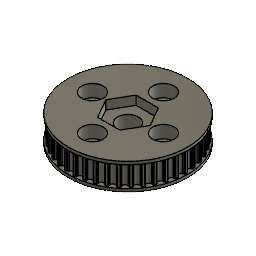
grt_cardan_joint_pulley_42T_20190328 (Autodesk Fusion 360 design; units mm, degrees)
Autodesk Fusion 360 part; units mm, degrees
(part 1 of 2)
sketch "Skizze1" plane through (0, 0, 0) normal (0, 1, 0) x (1, 0, 0)
  line L0 (0, 20.9325) -> (0, 0) construction
  arc A0 (-0.7739, 19.0309) -> (0, 18.5325) centre (0, 19.3825) ccw
  arc A1 (-0.8921, 19.4273) -> (-0.7739, 19.0309) centre (0.61, 19.6597) ccw
  arc A2 (-0.8921, 19.4273) -> (-1.1539, 19.6387) centre (-1.1392, 19.3891) ccw
  arc A3 (0, 20.5515) -> (-1.5358, 20.4941) centre (0, 0) ccw construction
  arc A4 (-1.1539, 19.6387) -> (-1.4701, 19.6175) centre (0, 0) ccw
  arc A5 (0, 20.9325) -> (-1.5643, 20.874) centre (0, 0) ccw construction
  line L1 (0, 0) -> (-1.5643, 20.874) construction
  line L2 (-1.4701, 19.6175) -> (0, 0)
  line L3 (0, 18.5325) -> (0, 0)
  dimension "d2" = 1.14
  dimension "d4" = 0.85
  dimension "d5" = 1.52
  dimension "d6" = 0.25
  dimension "d7" = 0.61
  dimension "d8" = 0.381
  dimension "d12" = 1.26
  dimension "d19" = 4.286
  dimension "d23" = 19.6725
  dimension "d24" = 2.4
  measures "d4" radius of A0
  measures "d5" radius of A1
  measures "d6" radius of A2
  measures "d19" angle of L0 L1
  measures "d23" distance of L0.end
  measures "d24" distance of L0.end
extrude "Extrusion1" add sketch "Skizze1" along normal blind 7 makes body 1
mirror "Spiegeln1" about plane through (0, 0, -18.5325) normal (1, 0, 0) of bodies 1 makes body 2
combine "Kombinieren1" operation add target body 1 tool bodies 2
pattern_circular "C-Anordnung1" count 42 over 360 about axis through (0, 1.75, 0) along (0, 1, 0) of bodies 1 makes body 3 at (-0.9801, 2.3333, -13.0783) makes body 4 at (-4.4504, 0, -12.0378) makes body 5 at (-6.1948, 0, -11.2401) makes body 6 at (-6.6368, 0, -10.9849) makes body 7 at (-8.1999, 0, -9.873) makes body 8 at (-9.5798, 7, -8.5406) makes body 9 at (-10.7457, 0, -7.0175) makes body 10 at (-11.6716, 0, -5.3375) makes body 11 at (-12.6502, 0, -2.1648) makes body 12 at (-12.7263, 0, -1.6601) makes body 13 at (-12.8316, 0, 0.2552) makes body 14 at (-12.6502, 0, 2.1648) makes body 15 at (-11.6716, 0, 5.3375) makes body 16 at (-10.7457, 0, 7.0175) makes body 17 at (-9.5798, 0, 8.5406) makes body 18 at (-9.2327, 7, 8.9148) makes body 19 at (-7.8009, 0, 10.1912) makes body 20 at (-4.9254, 0, 11.8514) makes body 21 at (-4.4504, 0, 12.0378) makes body 22 at (-1.2134, 0, 12.7766) makes body 23 at (-0.7044, 0, 12.8148) makes body 24 at (1.2134, 0, 12.7766) makes body 25 at (4.4504, 0, 12.0378) makes body 26 at (4.9254, 0, 11.8514) makes body 27 at (6.6368, 0, 10.9849) makes body 28 at (9.2327, 0, 8.9148) makes body 29 at (10.4582, 0, 7.4391) makes body 30 at (10.7457, 0, 7.0175) makes body 31 at (11.6716, 7, 5.3375) makes body 32 at (12.3367, 0, 3.5383) makes body 33 at (12.7263, 0, 1.6601) makes body 34 at (12.8316, 0, -0.2552) makes body 35 at (12.6502, 0, -2.1648) makes body 36 at (11.6716, 0, -5.3375) makes body 37 at (11.4502, 0, -5.7973) makes body 38 at (10.4582, 0, -7.4391) makes body 39 at (9.2327, 0, -8.9148) makes body 40 at (7.8009, 0, -10.1912) makes body 41 at (6.1948, 0, -11.2401) makes body 42 at (4.4504, 0, -12.0378) makes body 43 at (0.9801, 2.3333, -13.0783)
combine "Kombinieren2" operation add target body 1 tool bodies 21 20 19 3 18 17 8 15 7 12 9 11 10 16 6 5 14 4 13 41 31 39 27 22 23 29 25 24 26 42 28 43 30 38 34 33 37 32 36 35 40
sketch "Skizze2" plane through (0, 7, 0) normal (0, 1, 0) x (-1, 0, 0)
  arc A0 (-1.786, -19.5913) -> (-1.1539, -19.6387) centre (0, 0) ccw
  arc A1 (-1.1539, -19.6387) -> (-0.8921, -19.4273) centre (-1.1392, -19.3891) ccw
  arc A2 (-0.7739, -19.0309) -> (-0.8921, -19.4273) centre (0.61, -19.6597) ccw
  arc A3 (0.7739, -19.0309) -> (-0.7739, -19.0309) centre (0, -19.3825) ccw
  arc A4 (0.8921, -19.4273) -> (0.7739, -19.0309) centre (-0.61, -19.6597) ccw
  arc A5 (0.8921, -19.4273) -> (1.1539, -19.6387) centre (1.1392, -19.3891) ccw
  arc A6 (1.1539, -19.6387) -> (1.786, -19.5913) centre (0, 0) ccw
  arc A7 (1.786, -19.5913) -> (2.0133, -19.3433) centre (1.7633, -19.3423) ccw
  arc A8 (2.0712, -18.9337) -> (2.0133, -19.3433) centre (3.5333, -19.3492) ccw
  arc A9 (3.6017, -18.703) -> (2.0712, -18.9337) centre (2.8888, -19.166) ccw
  arc A10 (3.7777, -19.0773) -> (3.6017, -18.703) centre (2.3269, -19.531) ccw
  arc A11 (3.7777, -19.0773) -> (4.068, -19.2473) centre (4.0163, -19.0027) ccw
  arc A12 (4.068, -19.2473) -> (4.686, -19.1063) centre (0, 0) ccw
  arc A13 (4.686, -19.1063) -> (4.8738, -18.8272) centre (4.6264, -18.8635) ccw
  arc A14 (4.87, -18.4136) -> (4.8738, -18.8272) centre (6.3777, -18.6064) ccw
  arc A15 (6.349, -17.9573) -> (4.87, -18.4136) centre (5.7131, -18.5214) ccw
  arc A16 (6.5788, -18.3012) -> (6.349, -17.9573) centre (5.2119, -18.966) ccw
  arc A17 (6.5788, -18.3012) -> (6.8912, -18.4261) centre (6.8036, -18.1919) ccw
  arc A18 (6.8912, -18.4261) -> (7.4813, -18.1945) centre (0, 0) ccw
  arc A19 (7.4813, -18.1945) -> (7.6254, -17.8905) centre (7.3862, -17.9632) ccw
  arc A20 (7.56, -17.4821) -> (7.6254, -17.8905) centre (9.0796, -17.4481) ccw
  arc A21 (8.9545, -16.8105) -> (7.56, -17.4821) centre (8.4098, -17.463) ccw
  arc A22 (9.233, -17.1163) -> (8.9545, -16.8105) centre (7.9804, -17.9774) ccw
  arc A23 (9.233, -17.1163) -> (9.5605, -17.1932) centre (9.439, -16.9747) ccw
  arc A24 (9.5605, -17.1932) -> (10.1095, -16.8762) centre (0, 0) ccw
  arc A25 (10.1095, -16.8762) -> (10.2067, -16.5541) centre (9.981, -16.6617) ccw
  arc A26 (10.0811, -16.16) -> (10.2067, -16.5541) centre (11.5787, -15.8999) ccw
  arc A27 (11.3599, -15.2882) -> (10.0811, -16.16) centre (10.9186, -16.0146) ccw
  arc A28 (11.6809, -15.549) -> (11.3599, -15.2882) centre (10.5707, -16.5872) ccw
  arc A29 (11.6809, -15.549) -> (12.0162, -15.5762) centre (11.8635, -15.3783) ccw
  arc A30 (12.0162, -15.5762) -> (12.5118, -15.181) centre (0, 0) ccw
  arc A31 (12.5118, -15.181) -> (12.5599, -14.848) centre (12.3528, -14.9881) ccw
  arc A32 (12.377, -14.477) -> (12.5599, -14.848) centre (13.8191, -13.9966) ccw
  arc A33 (13.5116, -13.4243) -> (12.377, -14.477) centre (13.1835, -14.2084) ccw
  arc A34 (13.8679, -13.6344) -> (13.5116, -13.4243) centre (12.9248, -14.8264) ccw
  arc A35 (13.8679, -13.6344) -> (14.2035, -13.6113) centre (14.023, -13.4384) ccw
  arc A36 (14.2035, -13.6113) -> (14.6347, -13.1466) centre (0, 0) ccw
  arc A37 (14.6347, -13.1466) -> (14.6326, -12.8102) centre (14.4487, -12.9796) ccw
  arc A38 (14.3965, -12.4706) -> (14.6326, -12.8102) centre (15.7509, -11.7807) ccw
  arc A39 (15.3615, -11.2606) -> (14.3965, -12.4706) centre (15.1539, -12.0848) ccw
  arc A40 (15.7451, -11.4152) -> (15.3615, -11.2606) centre (14.9902, -12.7345) ccw
  arc A41 (15.7451, -11.4152) -> (16.0735, -11.3424) centre (15.8693, -11.1982) ccw
  arc A42 (16.0735, -11.3424) -> (16.4306, -10.8186) centre (0, 0) ccw
  arc A43 (16.4306, -10.8186) -> (16.3785, -10.4863) centre (16.2218, -10.6811) ccw
  arc A44 (16.0943, -10.1857) -> (16.3785, -10.4863) centre (17.3308, -9.3015) ccw
  arc A45 (16.8682, -8.8453) -> (16.0943, -10.1857) centre (16.7858, -9.6913) ccw
  arc A46 (17.2706, -8.941) -> (16.8682, -8.8453) centre (16.7208, -10.3581) ccw
  arc A47 (17.2706, -8.941) -> (17.5845, -8.8201) centre (17.361, -8.708) ccw
  arc A48 (17.5845, -8.8201) -> (17.8596, -8.2489) centre (0, 0) ccw
  arc A49 (17.8596, -8.2489) -> (17.7584, -7.9281) centre (17.6326, -8.1441) ccw
  arc A50 (17.4327, -7.6732) -> (17.7584, -7.9281) centre (18.5235, -6.6146) ccw
  arc A51 (17.9981, -6.2324) -> (17.4327, -7.6732) centre (18.0427, -7.0812) ccw
  arc A52 (18.4103, -6.2671) -> (17.9981, -6.2324) centre (18.0778, -7.7503) ccw
  arc A53 (18.4103, -6.2671) -> (18.7027, -6.1007) centre (18.465, -6.0232) ccw
  arc A54 (18.7027, -6.1007) -> (18.8895, -5.4949) centre (0, 0) ccw
  arc A55 (18.8895, -5.4949) -> (18.7417, -5.1927) centre (18.6495, -5.4251) ccw
  arc A56 (18.3816, -4.9893) -> (18.7417, -5.1927) centre (19.3025, -3.78) ccw
  arc A57 (18.726, -3.4803) -> (18.3816, -4.9893) centre (18.8966, -4.313) ccw
  arc A58 (19.1387, -3.4532) -> (18.726, -3.4803) centre (19.031, -4.9694) ccw
  arc A59 (19.1387, -3.4532) -> (19.403, -3.2451) centre (19.1565, -3.2038) ccw
  arc A60 (19.403, -3.2451) -> (19.4975, -2.6182) centre (0, 0) ccw
  arc A61 (19.4975, -2.6182) -> (19.3063, -2.3414) centre (19.2497, -2.585) ccw
  arc A62 (18.9199, -2.1939) -> (19.3063, -2.3414) centre (19.6503, -0.8609) ccw
  arc A63 (19.0356, -0.6505) -> (18.9199, -2.1939) centre (19.3283, -1.4485) ccw
  arc A64 (19.4396, -0.5622) -> (19.0356, -0.6505) centre (19.5591, -2.0775) ccw
  arc A65 (19.4396, -0.5622) -> (19.67, -0.317) centre (19.42, -0.3129) ccw
  arc A66 (19.67, -0.317) -> (19.67, 0.317) centre (0, 0) ccw
  arc A67 (19.67, 0.317) -> (19.4396, 0.5622) centre (19.42, 0.3129) ccw
  arc A68 (19.0356, 0.6505) -> (19.4396, 0.5622) centre (19.5591, 2.0775) ccw
  arc A69 (18.9199, 2.1939) -> (19.0356, 0.6505) centre (19.3283, 1.4485) ccw
  arc A70 (19.3063, 2.3414) -> (18.9199, 2.1939) centre (19.6503, 0.8609) ccw
  arc A71 (19.3063, 2.3414) -> (19.4975, 2.6182) centre (19.2497, 2.585) ccw
  arc A72 (19.4975, 2.6182) -> (19.403, 3.2451) centre (0, 0) ccw
  arc A73 (19.403, 3.2451) -> (19.1387, 3.4532) centre (19.1565, 3.2038) ccw
  arc A74 (18.726, 3.4803) -> (19.1387, 3.4532) centre (19.031, 4.9694) ccw
  arc A75 (18.3816, 4.9893) -> (18.726, 3.4803) centre (18.8966, 4.313) ccw
  arc A76 (18.7417, 5.1927) -> (18.3816, 4.9893) centre (19.3025, 3.78) ccw
  arc A77 (18.7417, 5.1927) -> (18.8895, 5.4949) centre (18.6495, 5.4251) ccw
  arc A78 (18.8895, 5.4949) -> (18.7027, 6.1007) centre (0, 0) ccw
  arc A79 (18.7027, 6.1007) -> (18.4103, 6.2671) centre (18.465, 6.0232) ccw
  arc A80 (17.9981, 6.2324) -> (18.4103, 6.2671) centre (18.0778, 7.7503) ccw
  arc A81 (17.4327, 7.6732) -> (17.9981, 6.2324) centre (18.0427, 7.0812) ccw
  arc A82 (17.7584, 7.9281) -> (17.4327, 7.6732) centre (18.5235, 6.6146) ccw
  arc A83 (17.7584, 7.9281) -> (17.8596, 8.2489) centre (17.6326, 8.1441) ccw
  arc A84 (17.8596, 8.2489) -> (17.5845, 8.8201) centre (0, 0) ccw
  arc A85 (17.5845, 8.8201) -> (17.2706, 8.941) centre (17.361, 8.708) ccw
  arc A86 (16.8682, 8.8453) -> (17.2706, 8.941) centre (16.7208, 10.3581) ccw
  arc A87 (16.0943, 10.1857) -> (16.8682, 8.8453) centre (16.7858, 9.6913) ccw
  arc A88 (16.3785, 10.4863) -> (16.0943, 10.1857) centre (17.3308, 9.3015) ccw
  arc A89 (16.3785, 10.4863) -> (16.4306, 10.8186) centre (16.2218, 10.6811) ccw
  arc A90 (16.4306, 10.8186) -> (16.0735, 11.3424) centre (0, 0) ccw
  arc A91 (16.0735, 11.3424) -> (15.7451, 11.4152) centre (15.8693, 11.1982) ccw
  arc A92 (15.3615, 11.2606) -> (15.7451, 11.4152) centre (14.9902, 12.7345) ccw
  arc A93 (14.3965, 12.4706) -> (15.3615, 11.2606) centre (15.1539, 12.0848) ccw
  arc A94 (14.6326, 12.8102) -> (14.3965, 12.4706) centre (15.7509, 11.7807) ccw
  arc A95 (14.6326, 12.8102) -> (14.6347, 13.1466) centre (14.4487, 12.9796) ccw
  arc A96 (14.6347, 13.1466) -> (14.2035, 13.6113) centre (0, 0) ccw
  arc A97 (14.2035, 13.6113) -> (13.8679, 13.6344) centre (14.023, 13.4384) ccw
  arc A98 (13.5116, 13.4243) -> (13.8679, 13.6344) centre (12.9248, 14.8264) ccw
  arc A99 (12.377, 14.477) -> (13.5116, 13.4243) centre (13.1835, 14.2084) ccw
  arc A100 (12.5599, 14.848) -> (12.377, 14.477) centre (13.8191, 13.9966) ccw
  arc A101 (12.5599, 14.848) -> (12.5118, 15.181) centre (12.3528, 14.9881) ccw
  arc A102 (12.5118, 15.181) -> (12.0162, 15.5762) centre (0, 0) ccw
  arc A103 (12.0162, 15.5762) -> (11.6809, 15.549) centre (11.8635, 15.3783) ccw
  arc A104 (11.3599, 15.2882) -> (11.6809, 15.549) centre (10.5707, 16.5872) ccw
  arc A105 (10.0811, 16.16) -> (11.3599, 15.2882) centre (10.9186, 16.0146) ccw
  arc A106 (10.2067, 16.5541) -> (10.0811, 16.16) centre (11.5787, 15.8999) ccw
  arc A107 (10.2067, 16.5541) -> (10.1095, 16.8762) centre (9.981, 16.6617) ccw
  arc A108 (10.1095, 16.8762) -> (9.5605, 17.1932) centre (0, 0) ccw
  arc A109 (9.5605, 17.1932) -> (9.233, 17.1163) centre (9.439, 16.9747) ccw
  arc A110 (8.9545, 16.8105) -> (9.233, 17.1163) centre (7.9804, 17.9774) ccw
  arc A111 (7.56, 17.4821) -> (8.9545, 16.8105) centre (8.4098, 17.463) ccw
  arc A112 (7.6254, 17.8905) -> (7.56, 17.4821) centre (9.0796, 17.4481) ccw
  arc A113 (7.6254, 17.8905) -> (7.4813, 18.1945) centre (7.3862, 17.9632) ccw
  arc A114 (7.4813, 18.1945) -> (6.8912, 18.4261) centre (0, 0) ccw
  arc A115 (6.8912, 18.4261) -> (6.5788, 18.3012) centre (6.8036, 18.1919) ccw
  arc A116 (6.349, 17.9573) -> (6.5788, 18.3012) centre (5.2119, 18.966) ccw
  arc A117 (4.87, 18.4136) -> (6.349, 17.9573) centre (5.7131, 18.5214) ccw
  arc A118 (4.8738, 18.8272) -> (4.87, 18.4136) centre (6.3777, 18.6064) ccw
  arc A119 (4.8738, 18.8272) -> (4.686, 19.1063) centre (4.6264, 18.8635) ccw
  arc A120 (4.686, 19.1063) -> (4.068, 19.2473) centre (0, 0) ccw
  arc A121 (4.068, 19.2473) -> (3.7777, 19.0773) centre (4.0163, 19.0027) ccw
  arc A122 (3.6017, 18.703) -> (3.7777, 19.0773) centre (2.3269, 19.531) ccw
  arc A123 (2.0712, 18.9337) -> (3.6017, 18.703) centre (2.8888, 19.166) ccw
  arc A124 (2.0133, 19.3433) -> (2.0712, 18.9337) centre (3.5333, 19.3492) ccw
  arc A125 (2.0133, 19.3433) -> (1.786, 19.5913) centre (1.7633, 19.3423) ccw
  arc A126 (1.786, 19.5913) -> (1.1539, 19.6387) centre (0, 0) ccw
  arc A127 (1.1539, 19.6387) -> (0.8921, 19.4273) centre (1.1392, 19.3891) ccw
  arc A128 (0.7739, 19.0309) -> (0.8921, 19.4273) centre (-0.61, 19.6597) ccw
  arc A129 (-0.7739, 19.0309) -> (0.7739, 19.0309) centre (0, 19.3825) ccw
  arc A130 (-0.8921, 19.4273) -> (-0.7739, 19.0309) centre (0.61, 19.6597) ccw
  arc A131 (-0.8921, 19.4273) -> (-1.1539, 19.6387) centre (-1.1392, 19.3891) ccw
  arc A132 (-1.1539, 19.6387) -> (-1.786, 19.5913) centre (0, 0) ccw
  arc A133 (-1.786, 19.5913) -> (-2.0133, 19.3433) centre (-1.7633, 19.3423) ccw
  arc A134 (-2.0712, 18.9337) -> (-2.0133, 19.3433) centre (-3.5333, 19.3492) ccw
  arc A135 (-3.6017, 18.703) -> (-2.0712, 18.9337) centre (-2.8888, 19.166) ccw
  arc A136 (-3.7777, 19.0773) -> (-3.6017, 18.703) centre (-2.3269, 19.531) ccw
  arc A137 (-3.7777, 19.0773) -> (-4.068, 19.2473) centre (-4.0163, 19.0027) ccw
  arc A138 (-4.068, 19.2473) -> (-4.686, 19.1063) centre (0, 0) ccw
  arc A139 (-4.686, 19.1063) -> (-4.8738, 18.8272) centre (-4.6264, 18.8635) ccw
  arc A140 (-4.87, 18.4136) -> (-4.8738, 18.8272) centre (-6.3777, 18.6064) ccw
  arc A141 (-6.349, 17.9573) -> (-4.87, 18.4136) centre (-5.7131, 18.5214) ccw
  arc A142 (-6.5788, 18.3012) -> (-6.349, 17.9573) centre (-5.2119, 18.966) ccw
  arc A143 (-6.5788, 18.3012) -> (-6.8912, 18.4261) centre (-6.8036, 18.1919) ccw
  arc A144 (-6.8912, 18.4261) -> (-7.4813, 18.1945) centre (0, 0) ccw
  arc A145 (-7.4813, 18.1945) -> (-7.6254, 17.8905) centre (-7.3862, 17.9632) ccw
  arc A146 (-7.56, 17.4821) -> (-7.6254, 17.8905) centre (-9.0796, 17.4481) ccw
  arc A147 (-8.9545, 16.8105) -> (-7.56, 17.4821) centre (-8.4098, 17.463) ccw
  arc A148 (-9.233, 17.1163) -> (-8.9545, 16.8105) centre (-7.9804, 17.9774) ccw
  arc A149 (-9.233, 17.1163) -> (-9.5605, 17.1932) centre (-9.439, 16.9747) ccw
  arc A150 (-9.5605, 17.1932) -> (-10.1095, 16.8762) centre (0, 0) ccw
  arc A151 (-10.1095, 16.8762) -> (-10.2067, 16.5541) centre (-9.981, 16.6617) ccw
  arc A152 (-10.0811, 16.16) -> (-10.2067, 16.5541) centre (-11.5787, 15.8999) ccw
  arc A153 (-11.3599, 15.2882) -> (-10.0811, 16.16) centre (-10.9186, 16.0146) ccw
  arc A154 (-11.6809, 15.549) -> (-11.3599, 15.2882) centre (-10.5707, 16.5872) ccw
  arc A155 (-11.6809, 15.549) -> (-12.0162, 15.5762) centre (-11.8635, 15.3783) ccw
  arc A156 (-12.0162, 15.5762) -> (-12.5118, 15.181) centre (0, 0) ccw
  arc A157 (-12.5118, 15.181) -> (-12.5599, 14.848) centre (-12.3528, 14.9881) ccw
  arc A158 (-12.377, 14.477) -> (-12.5599, 14.848) centre (-13.8191, 13.9966) ccw
  arc A159 (-13.5116, 13.4243) -> (-12.377, 14.477) centre (-13.1835, 14.2084) ccw
  arc A160 (-13.8679, 13.6344) -> (-13.5116, 13.4243) centre (-12.9248, 14.8264) ccw
  arc A161 (-13.8679, 13.6344) -> (-14.2035, 13.6113) centre (-14.023, 13.4384) ccw
  arc A162 (-14.2035, 13.6113) -> (-14.6347, 13.1466) centre (0, 0) ccw
  arc A163 (-14.6347, 13.1466) -> (-14.6326, 12.8102) centre (-14.4487, 12.9796) ccw
  arc A164 (-14.3965, 12.4706) -> (-14.6326, 12.8102) centre (-15.7509, 11.7807) ccw
  arc A165 (-15.3615, 11.2606) -> (-14.3965, 12.4706) centre (-15.1539, 12.0848) ccw
  arc A166 (-15.7451, 11.4152) -> (-15.3615, 11.2606) centre (-14.9902, 12.7345) ccw
  arc A167 (-15.7451, 11.4152) -> (-16.0735, 11.3424) centre (-15.8693, 11.1982) ccw
  arc A168 (-16.0735, 11.3424) -> (-16.4306, 10.8186) centre (0, 0) ccw
  arc A169 (-16.4306, 10.8186) -> (-16.3785, 10.4863) centre (-16.2218, 10.6811) ccw
  arc A170 (-16.0943, 10.1857) -> (-16.3785, 10.4863) centre (-17.3308, 9.3015) ccw
  arc A171 (-16.8682, 8.8453) -> (-16.0943, 10.1857) centre (-16.7858, 9.6913) ccw
  arc A172 (-17.2706, 8.941) -> (-16.8682, 8.8453) centre (-16.7208, 10.3581) ccw
  arc A173 (-17.2706, 8.941) -> (-17.5845, 8.8201) centre (-17.361, 8.708) ccw
  arc A174 (-17.5845, 8.8201) -> (-17.8596, 8.2489) centre (0, 0) ccw
  arc A175 (-17.8596, 8.2489) -> (-17.7584, 7.9281) centre (-17.6326, 8.1441) ccw
  arc A176 (-17.4327, 7.6732) -> (-17.7584, 7.9281) centre (-18.5235, 6.6146) ccw
  arc A177 (-17.9981, 6.2324) -> (-17.4327, 7.6732) centre (-18.0427, 7.0812) ccw
  arc A178 (-18.4103, 6.2671) -> (-17.9981, 6.2324) centre (-18.0778, 7.7503) ccw
  arc A179 (-18.4103, 6.2671) -> (-18.7027, 6.1007) centre (-18.465, 6.0232) ccw
  arc A180 (-18.7027, 6.1007) -> (-18.8895, 5.4949) centre (0, 0) ccw
  arc A181 (-18.8895, 5.4949) -> (-18.7417, 5.1927) centre (-18.6495, 5.4251) ccw
  arc A182 (-18.3816, 4.9893) -> (-18.7417, 5.1927) centre (-19.3025, 3.78) ccw
  arc A183 (-18.726, 3.4803) -> (-18.3816, 4.9893) centre (-18.8966, 4.313) ccw
  arc A184 (-19.1387, 3.4532) -> (-18.726, 3.4803) centre (-19.031, 4.9694) ccw
  arc A185 (-19.1387, 3.4532) -> (-19.403, 3.2451) centre (-19.1565, 3.2038) ccw
  arc A186 (-19.403, 3.2451) -> (-19.4975, 2.6182) centre (0, 0) ccw
  arc A187 (-19.4975, 2.6182) -> (-19.3063, 2.3414) centre (-19.2497, 2.585) ccw
  arc A188 (-18.9199, 2.1939) -> (-19.3063, 2.3414) centre (-19.6503, 0.8609) ccw
  arc A189 (-19.0356, 0.6505) -> (-18.9199, 2.1939) centre (-19.3283, 1.4485) ccw
  arc A190 (-19.4396, 0.5622) -> (-19.0356, 0.6505) centre (-19.5591, 2.0775) ccw
  arc A191 (-19.4396, 0.5622) -> (-19.67, 0.317) centre (-19.42, 0.3129) ccw
  arc A192 (-19.67, 0.317) -> (-19.67, -0.317) centre (0, 0) ccw
  arc A193 (-19.67, -0.317) -> (-19.4396, -0.5622) centre (-19.42, -0.3129) ccw
  arc A194 (-19.0356, -0.6505) -> (-19.4396, -0.5622) centre (-19.5591, -2.0775) ccw
  arc A195 (-18.9199, -2.1939) -> (-19.0356, -0.6505) centre (-19.3283, -1.4485) ccw
  arc A196 (-19.3063, -2.3414) -> (-18.9199, -2.1939) centre (-19.6503, -0.8609) ccw
  arc A197 (-19.3063, -2.3414) -> (-19.4975, -2.6182) centre (-19.2497, -2.585) ccw
  arc A198 (-19.4975, -2.6182) -> (-19.403, -3.2451) centre (0, 0) ccw
  arc A199 (-19.403, -3.2451) -> (-19.1387, -3.4532) centre (-19.1565, -3.2038) ccw
  arc A200 (-18.726, -3.4803) -> (-19.1387, -3.4532) centre (-19.031, -4.9694) ccw
  arc A201 (-18.3816, -4.9893) -> (-18.726, -3.4803) centre (-18.8966, -4.313) ccw
  arc A202 (-18.7417, -5.1927) -> (-18.3816, -4.9893) centre (-19.3025, -3.78) ccw
  arc A203 (-18.7417, -5.1927) -> (-18.8895, -5.4949) centre (-18.6495, -5.4251) ccw
  arc A204 (-18.8895, -5.4949) -> (-18.7027, -6.1007) centre (0, 0) ccw
  arc A205 (-18.7027, -6.1007) -> (-18.4103, -6.2671) centre (-18.465, -6.0232) ccw
  arc A206 (-17.9981, -6.2324) -> (-18.4103, -6.2671) centre (-18.0778, -7.7503) ccw
  arc A207 (-17.4327, -7.6732) -> (-17.9981, -6.2324) centre (-18.0427, -7.0812) ccw
  arc A208 (-17.7584, -7.9281) -> (-17.4327, -7.6732) centre (-18.5235, -6.6146) ccw
  arc A209 (-17.7584, -7.9281) -> (-17.8596, -8.2489) centre (-17.6326, -8.1441) ccw
  arc A210 (-17.8596, -8.2489) -> (-17.5845, -8.8201) centre (0, 0) ccw
  arc A211 (-17.5845, -8.8201) -> (-17.2706, -8.941) centre (-17.361, -8.708) ccw
  arc A212 (-16.8682, -8.8453) -> (-17.2706, -8.941) centre (-16.7208, -10.3581) ccw
  arc A213 (-16.0943, -10.1857) -> (-16.8682, -8.8453) centre (-16.7858, -9.6913) ccw
  arc A214 (-16.3785, -10.4863) -> (-16.0943, -10.1857) centre (-17.3308, -9.3015) ccw
  arc A215 (-16.3785, -10.4863) -> (-16.4306, -10.8186) centre (-16.2218, -10.6811) ccw
  arc A216 (-16.4306, -10.8186) -> (-16.0735, -11.3424) centre (0, 0) ccw
  arc A217 (-16.0735, -11.3424) -> (-15.7451, -11.4152) centre (-15.8693, -11.1982) ccw
  arc A218 (-15.3615, -11.2606) -> (-15.7451, -11.4152) centre (-14.9902, -12.7345) ccw
  arc A219 (-14.3965, -12.4706) -> (-15.3615, -11.2606) centre (-15.1539, -12.0848) ccw
  arc A220 (-14.6326, -12.8102) -> (-14.3965, -12.4706) centre (-15.7509, -11.7807) ccw
  arc A221 (-14.6326, -12.8102) -> (-14.6347, -13.1466) centre (-14.4487, -12.9796) ccw
  arc A222 (-14.6347, -13.1466) -> (-14.2035, -13.6113) centre (0, 0) ccw
  arc A223 (-14.2035, -13.6113) -> (-13.8679, -13.6344) centre (-14.023, -13.4384) ccw
  arc A224 (-13.5116, -13.4243) -> (-13.8679, -13.6344) centre (-12.9248, -14.8264) ccw
  arc A225 (-12.377, -14.477) -> (-13.5116, -13.4243) centre (-13.1835, -14.2084) ccw
  arc A226 (-12.5599, -14.848) -> (-12.377, -14.477) centre (-13.8191, -13.9966) ccw
  arc A227 (-12.5599, -14.848) -> (-12.5118, -15.181) centre (-12.3528, -14.9881) ccw
  arc A228 (-12.5118, -15.181) -> (-12.0162, -15.5762) centre (0, 0) ccw
  arc A229 (-12.0162, -15.5762) -> (-11.6809, -15.549) centre (-11.8635, -15.3783) ccw
  arc A230 (-11.3599, -15.2882) -> (-11.6809, -15.549) centre (-10.5707, -16.5872) ccw
  arc A231 (-10.0811, -16.16) -> (-11.3599, -15.2882) centre (-10.9186, -16.0146) ccw
  arc A232 (-10.2067, -16.5541) -> (-10.0811, -16.16) centre (-11.5787, -15.8999) ccw
  arc A233 (-10.2067, -16.5541) -> (-10.1095, -16.8762) centre (-9.981, -16.6617) ccw
  arc A234 (-10.1095, -16.8762) -> (-9.5605, -17.1932) centre (0, 0) ccw
  arc A235 (-9.5605, -17.1932) -> (-9.233, -17.1163) centre (-9.439, -16.9747) ccw
  arc A236 (-8.9545, -16.8105) -> (-9.233, -17.1163) centre (-7.9804, -17.9774) ccw
  arc A237 (-7.56, -17.4821) -> (-8.9545, -16.8105) centre (-8.4098, -17.463) ccw
  arc A238 (-7.6254, -17.8905) -> (-7.56, -17.4821) centre (-9.0796, -17.4481) ccw
  arc A239 (-7.6254, -17.8905) -> (-7.4813, -18.1945) centre (-7.3862, -17.9632) ccw
  circle A240 centre (0, 0) radius 20.6725
  arc A241 (-7.4813, -18.1945) -> (-6.8912, -18.4261) centre (0, 0) ccw
  arc A242 (-6.8912, -18.4261) -> (-6.5788, -18.3012) centre (-6.8036, -18.1919) ccw
  arc A243 (-6.349, -17.9573) -> (-6.5788, -18.3012) centre (-5.2119, -18.966) ccw
  arc A244 (-4.87, -18.4136) -> (-6.349, -17.9573) centre (-5.7131, -18.5214) ccw
  arc A245 (-4.8738, -18.8272) -> (-4.87, -18.4136) centre (-6.3777, -18.6064) ccw
  arc A246 (-4.8738, -18.8272) -> (-4.686, -19.1063) centre (-4.6264, -18.8635) ccw
  arc A247 (-4.686, -19.1063) -> (-4.068, -19.2473) centre (0, 0) ccw
  arc A248 (-4.068, -19.2473) -> (-3.7777, -19.0773) centre (-4.0163, -19.0027) ccw
  arc A249 (-3.6017, -18.703) -> (-3.7777, -19.0773) centre (-2.3269, -19.531) ccw
  arc A250 (-2.0712, -18.9337) -> (-3.6017, -18.703) centre (-2.8888, -19.166) ccw
  arc A251 (-2.0133, -19.3433) -> (-2.0712, -18.9337) centre (-3.5333, -19.3492) ccw
  arc A252 (-2.0133, -19.3433) -> (-1.786, -19.5913) centre (-1.7633, -19.3423) ccw
  dimension "d30" = 41.345
  measures "d30" diameter of A240
extrude "Extrusion2" add sketch "Skizze2" along normal blind 1 contours A0 A1 A2 A3 A4 A5 A6 A7 A8 A9 A10 A11 A12 A13 A14 A15 A16 A17 A18 A19 A20 A21 A22 A23 A24 A25 A26 A27 A28 A29 A30 A31 A32 A33 A34 A35 A36 A37 A38 A39 A40 A41 A42 A43 A44 A45 A46 A47 A48 A49 A50 A51 A52 A53 A54 A55 A56 A57 A58 A59 A60 A61 A62 A63 A64 A65 A66 A67 A68 A69 A70 A71 A72 A73 A74 A75 A76 A77 A78 A79 A80 A81 A82 A83 A84 A85 A86 A87 A88 A89 A90 A91 A92 A93 A94 A95 A96 A97 A98 A99 A100 A101 A102 A103 A104 A105 A106 A107 A108 A109 A110 A111 A112 A113 A114 A115 A116 A117 A118 A119 A120 A121 A122 A123 A124 A125 A126 A127 A128 A129 A130 A131 A132 A133 A134 A135 A136 A137 A138 A139 A140 A141 A142 A143 A144 A145 A146 A147 A148 A149 A150 A151 A152 A153 A154 A155 A156 A157 A158 A159 A160 A161 A162 A163 A164 A165 A166 A167 A168 A169 A170 A171 A172 A173 A174 A175 A176 A177 A178 A179 A180 A181 A182 A183 A184 A185 A186 A187 A188 A189 A190 A191 A192 A193 A194 A195 A196 A197 A198 A199 A200 A201 A202 A203 A204 A205 A206 A207 A208 A209 A210 A211 A212 A213 A214 A215 A216 A217 A218 A219 A220 A221 A222 A223 A224 A225 A226 A227 A228 A229 A230 A231 A232 A233 A234 A235 A236 A237 A238 A239 A241 A242 A243 A244 A245 A246 A247 A248 A249 A250 A251 A252 | A240 bodies 1
sketch "Skizze3" plane through (0, 0, 0) normal (0, -1, 0) x (1, 0, 0)
  arc A0 (7.4813, -18.1945) -> (7.6254, -17.8905) centre (7.3862, -17.9632) ccw
  arc A1 (7.56, -17.4821) -> (7.6254, -17.8905) centre (9.0796, -17.4481) ccw
  arc A2 (8.9545, -16.8105) -> (7.56, -17.4821) centre (8.4098, -17.463) ccw
  arc A3 (9.233, -17.1163) -> (8.9545, -16.8105) centre (7.9804, -17.9774) ccw
  arc A4 (9.233, -17.1163) -> (9.5605, -17.1932) centre (9.439, -16.9747) ccw
  arc A5 (9.5605, -17.1932) -> (10.1095, -16.8762) centre (0, 0) ccw
  arc A6 (10.1095, -16.8762) -> (10.2067, -16.5541) centre (9.981, -16.6617) ccw
  arc A7 (10.0811, -16.16) -> (10.2067, -16.5541) centre (11.5787, -15.8999) ccw
  arc A8 (11.3599, -15.2882) -> (10.0811, -16.16) centre (10.9186, -16.0146) ccw
  arc A9 (11.6809, -15.549) -> (11.3599, -15.2882) centre (10.5707, -16.5872) ccw
  arc A10 (11.6809, -15.549) -> (12.0162, -15.5762) centre (11.8635, -15.3783) ccw
  arc A11 (12.0162, -15.5762) -> (12.5118, -15.181) centre (0, 0) ccw
  arc A12 (12.5118, -15.181) -> (12.5599, -14.848) centre (12.3528, -14.9881) ccw
  arc A13 (12.377, -14.477) -> (12.5599, -14.848) centre (13.8191, -13.9966) ccw
  arc A14 (13.5116, -13.4243) -> (12.377, -14.477) centre (13.1835, -14.2084) ccw
  arc A15 (13.8679, -13.6344) -> (13.5116, -13.4243) centre (12.9248, -14.8264) ccw
  arc A16 (13.8679, -13.6344) -> (14.2035, -13.6113) centre (14.023, -13.4384) ccw
  arc A17 (14.2035, -13.6113) -> (14.6347, -13.1466) centre (0, 0) ccw
  arc A18 (14.6347, -13.1466) -> (14.6326, -12.8102) centre (14.4487, -12.9796) ccw
  arc A19 (14.3965, -12.4706) -> (14.6326, -12.8102) centre (15.7509, -11.7807) ccw
  arc A20 (15.3615, -11.2606) -> (14.3965, -12.4706) centre (15.1539, -12.0848) ccw
  arc A21 (15.7451, -11.4152) -> (15.3615, -11.2606) centre (14.9902, -12.7345) ccw
  arc A22 (15.7451, -11.4152) -> (16.0735, -11.3424) centre (15.8693, -11.1982) ccw
  arc A23 (16.0735, -11.3424) -> (16.4306, -10.8186) centre (0, 0) ccw
  arc A24 (16.4306, -10.8186) -> (16.3785, -10.4863) centre (16.2218, -10.6811) ccw
  arc A25 (16.0943, -10.1857) -> (16.3785, -10.4863) centre (17.3308, -9.3015) ccw
  arc A26 (16.8682, -8.8453) -> (16.0943, -10.1857) centre (16.7858, -9.6913) ccw
  arc A27 (17.2706, -8.941) -> (16.8682, -8.8453) centre (16.7208, -10.3581) ccw
  arc A28 (17.2706, -8.941) -> (17.5845, -8.8201) centre (17.361, -8.708) ccw
  arc A29 (17.5845, -8.8201) -> (17.8596, -8.2489) centre (0, 0) ccw
  arc A30 (17.8596, -8.2489) -> (17.7584, -7.9281) centre (17.6326, -8.1441) ccw
  arc A31 (17.4327, -7.6732) -> (17.7584, -7.9281) centre (18.5235, -6.6146) ccw
  arc A32 (17.9981, -6.2324) -> (17.4327, -7.6732) centre (18.0427, -7.0812) ccw
  arc A33 (18.4103, -6.2671) -> (17.9981, -6.2324) centre (18.0778, -7.7503) ccw
  arc A34 (18.4103, -6.2671) -> (18.7027, -6.1007) centre (18.465, -6.0232) ccw
  arc A35 (18.7027, -6.1007) -> (18.8895, -5.4949) centre (0, 0) ccw
  arc A36 (18.8895, -5.4949) -> (18.7417, -5.1927) centre (18.6495, -5.4251) ccw
  arc A37 (18.3816, -4.9893) -> (18.7417, -5.1927) centre (19.3025, -3.78) ccw
  arc A38 (18.726, -3.4803) -> (18.3816, -4.9893) centre (18.8966, -4.313) ccw
  arc A39 (19.1387, -3.4532) -> (18.726, -3.4803) centre (19.031, -4.9694) ccw
  arc A40 (19.1387, -3.4532) -> (19.403, -3.2451) centre (19.1565, -3.2038) ccw
  arc A41 (19.403, -3.2451) -> (19.4975, -2.6182) centre (0, 0) ccw
  arc A42 (19.4975, -2.6182) -> (19.3063, -2.3414) centre (19.2497, -2.585) ccw
  arc A43 (18.9199, -2.1939) -> (19.3063, -2.3414) centre (19.6503, -0.8609) ccw
  arc A44 (19.0356, -0.6505) -> (18.9199, -2.1939) centre (19.3283, -1.4485) ccw
  arc A45 (19.4396, -0.5622) -> (19.0356, -0.6505) centre (19.5591, -2.0775) ccw
  arc A46 (19.4396, -0.5622) -> (19.67, -0.317) centre (19.42, -0.3129) ccw
  arc A47 (19.67, -0.317) -> (19.67, 0.317) centre (0, 0) ccw
  arc A48 (19.67, 0.317) -> (19.4396, 0.5622) centre (19.42, 0.3129) ccw
  arc A49 (19.0356, 0.6505) -> (19.4396, 0.5622) centre (19.5591, 2.0775) ccw
  arc A50 (18.9199, 2.1939) -> (19.0356, 0.6505) centre (19.3283, 1.4485) ccw
  arc A51 (19.3063, 2.3414) -> (18.9199, 2.1939) centre (19.6503, 0.8609) ccw
  arc A52 (19.3063, 2.3414) -> (19.4975, 2.6182) centre (19.2497, 2.585) ccw
  arc A53 (19.4975, 2.6182) -> (19.403, 3.2451) centre (0, 0) ccw
  arc A54 (19.403, 3.2451) -> (19.1387, 3.4532) centre (19.1565, 3.2038) ccw
  arc A55 (18.726, 3.4803) -> (19.1387, 3.4532) centre (19.031, 4.9694) ccw
  arc A56 (18.3816, 4.9893) -> (18.726, 3.4803) centre (18.8966, 4.313) ccw
  arc A57 (18.7417, 5.1927) -> (18.3816, 4.9893) centre (19.3025, 3.78) ccw
  arc A58 (18.7417, 5.1927) -> (18.8895, 5.4949) centre (18.6495, 5.4251) ccw
  arc A59 (18.8895, 5.4949) -> (18.7027, 6.1007) centre (0, 0) ccw
  arc A60 (18.7027, 6.1007) -> (18.4103, 6.2671) centre (18.465, 6.0232) ccw
  arc A61 (17.9981, 6.2324) -> (18.4103, 6.2671) centre (18.0778, 7.7503) ccw
  arc A62 (17.4327, 7.6732) -> (17.9981, 6.2324) centre (18.0427, 7.0812) ccw
  arc A63 (17.7584, 7.9281) -> (17.4327, 7.6732) centre (18.5235, 6.6146) ccw
  arc A64 (17.7584, 7.9281) -> (17.8596, 8.2489) centre (17.6326, 8.1441) ccw
  arc A65 (17.8596, 8.2489) -> (17.5845, 8.8201) centre (0, 0) ccw
  arc A66 (17.5845, 8.8201) -> (17.2706, 8.941) centre (17.361, 8.708) ccw
  arc A67 (16.8682, 8.8453) -> (17.2706, 8.941) centre (16.7208, 10.3581) ccw
  arc A68 (16.0943, 10.1857) -> (16.8682, 8.8453) centre (16.7858, 9.6913) ccw
  arc A69 (16.3785, 10.4863) -> (16.0943, 10.1857) centre (17.3308, 9.3015) ccw
  arc A70 (16.3785, 10.4863) -> (16.4306, 10.8186) centre (16.2218, 10.6811) ccw
  arc A71 (16.4306, 10.8186) -> (16.0735, 11.3424) centre (0, 0) ccw
  arc A72 (16.0735, 11.3424) -> (15.7451, 11.4152) centre (15.8693, 11.1982) ccw
  arc A73 (15.3615, 11.2606) -> (15.7451, 11.4152) centre (14.9902, 12.7345) ccw
  arc A74 (14.3965, 12.4706) -> (15.3615, 11.2606) centre (15.1539, 12.0848) ccw
  arc A75 (14.6326, 12.8102) -> (14.3965, 12.4706) centre (15.7509, 11.7807) ccw
  arc A76 (14.6326, 12.8102) -> (14.6347, 13.1466) centre (14.4487, 12.9796) ccw
  arc A77 (14.6347, 13.1466) -> (14.2035, 13.6113) centre (0, 0) ccw
  arc A78 (14.2035, 13.6113) -> (13.8679, 13.6344) centre (14.023, 13.4384) ccw
  arc A79 (13.5116, 13.4243) -> (13.8679, 13.6344) centre (12.9248, 14.8264) ccw
  arc A80 (12.377, 14.477) -> (13.5116, 13.4243) centre (13.1835, 14.2084) ccw
  arc A81 (12.5599, 14.848) -> (12.377, 14.477) centre (13.8191, 13.9966) ccw
  arc A82 (12.5599, 14.848) -> (12.5118, 15.181) centre (12.3528, 14.9881) ccw
  arc A83 (12.5118, 15.181) -> (12.0162, 15.5762) centre (0, 0) ccw
  arc A84 (12.0162, 15.5762) -> (11.6809, 15.549) centre (11.8635, 15.3783) ccw
  arc A85 (11.3599, 15.2882) -> (11.6809, 15.549) centre (10.5707, 16.5872) ccw
  arc A86 (10.0811, 16.16) -> (11.3599, 15.2882) centre (10.9186, 16.0146) ccw
  arc A87 (10.2067, 16.5541) -> (10.0811, 16.16) centre (11.5787, 15.8999) ccw
  arc A88 (10.2067, 16.5541) -> (10.1095, 16.8762) centre (9.981, 16.6617) ccw
  arc A89 (10.1095, 16.8762) -> (9.5605, 17.1932) centre (0, 0) ccw
  arc A90 (9.5605, 17.1932) -> (9.233, 17.1163) centre (9.439, 16.9747) ccw
  arc A91 (8.9545, 16.8105) -> (9.233, 17.1163) centre (7.9804, 17.9774) ccw
  arc A92 (7.56, 17.4821) -> (8.9545, 16.8105) centre (8.4098, 17.463) ccw
  arc A93 (7.6254, 17.8905) -> (7.56, 17.4821) centre (9.0796, 17.4481) ccw
  arc A94 (7.6254, 17.8905) -> (7.4813, 18.1945) centre (7.3862, 17.9632) ccw
  arc A95 (7.4813, 18.1945) -> (6.8912, 18.4261) centre (0, 0) ccw
  arc A96 (6.8912, 18.4261) -> (6.5788, 18.3012) centre (6.8036, 18.1919) ccw
  arc A97 (6.349, 17.9573) -> (6.5788, 18.3012) centre (5.2119, 18.966) ccw
  arc A98 (4.87, 18.4136) -> (6.349, 17.9573) centre (5.7131, 18.5214) ccw
  arc A99 (4.8738, 18.8272) -> (4.87, 18.4136) centre (6.3777, 18.6064) ccw
  arc A100 (4.8738, 18.8272) -> (4.686, 19.1063) centre (4.6264, 18.8635) ccw
  arc A101 (4.686, 19.1063) -> (4.068, 19.2473) centre (0, 0) ccw
  arc A102 (4.068, 19.2473) -> (3.7777, 19.0773) centre (4.0163, 19.0027) ccw
  arc A103 (3.6017, 18.703) -> (3.7777, 19.0773) centre (2.3269, 19.531) ccw
  arc A104 (2.0712, 18.9337) -> (3.6017, 18.703) centre (2.8888, 19.166) ccw
  arc A105 (2.0133, 19.3433) -> (2.0712, 18.9337) centre (3.5333, 19.3492) ccw
  arc A106 (2.0133, 19.3433) -> (1.786, 19.5913) centre (1.7633, 19.3423) ccw
  arc A107 (1.786, 19.5913) -> (1.1539, 19.6387) centre (0, 0) ccw
  arc A108 (1.1539, 19.6387) -> (0.8921, 19.4273) centre (1.1392, 19.3891) ccw
  arc A109 (0.7739, 19.0309) -> (0.8921, 19.4273) centre (-0.61, 19.6597) ccw
  arc A110 (-0.7739, 19.0309) -> (0.7739, 19.0309) centre (0, 19.3825) ccw
  arc A111 (-0.8921, 19.4273) -> (-0.7739, 19.0309) centre (0.61, 19.6597) ccw
  arc A112 (-0.8921, 19.4273) -> (-1.1539, 19.6387) centre (-1.1392, 19.3891) ccw
  arc A113 (-1.1539, 19.6387) -> (-1.786, 19.5913) centre (0, 0) ccw
  arc A114 (-1.786, 19.5913) -> (-2.0133, 19.3433) centre (-1.7633, 19.3423) ccw
  arc A115 (-2.0712, 18.9337) -> (-2.0133, 19.3433) centre (-3.5333, 19.3492) ccw
  arc A116 (-3.6017, 18.703) -> (-2.0712, 18.9337) centre (-2.8888, 19.166) ccw
  arc A117 (-3.7777, 19.0773) -> (-3.6017, 18.703) centre (-2.3269, 19.531) ccw
  arc A118 (-3.7777, 19.0773) -> (-4.068, 19.2473) centre (-4.0163, 19.0027) ccw
  arc A119 (-4.068, 19.2473) -> (-4.686, 19.1063) centre (0, 0) ccw
  arc A120 (-4.686, 19.1063) -> (-4.8738, 18.8272) centre (-4.6264, 18.8635) ccw
  arc A121 (-4.87, 18.4136) -> (-4.8738, 18.8272) centre (-6.3777, 18.6064) ccw
  arc A122 (-6.349, 17.9573) -> (-4.87, 18.4136) centre (-5.7131, 18.5214) ccw
  arc A123 (-6.5788, 18.3012) -> (-6.349, 17.9573) centre (-5.2119, 18.966) ccw
  arc A124 (-6.5788, 18.3012) -> (-6.8912, 18.4261) centre (-6.8036, 18.1919) ccw
  arc A125 (-6.8912, 18.4261) -> (-7.4813, 18.1945) centre (0, 0) ccw
  arc A126 (-7.4813, 18.1945) -> (-7.6254, 17.8905) centre (-7.3862, 17.9632) ccw
  arc A127 (-7.56, 17.4821) -> (-7.6254, 17.8905) centre (-9.0796, 17.4481) ccw
  arc A128 (-8.9545, 16.8105) -> (-7.56, 17.4821) centre (-8.4098, 17.463) ccw
  arc A129 (-9.233, 17.1163) -> (-8.9545, 16.8105) centre (-7.9804, 17.9774) ccw
  arc A130 (-9.233, 17.1163) -> (-9.5605, 17.1932) centre (-9.439, 16.9747) ccw
  arc A131 (-9.5605, 17.1932) -> (-10.1095, 16.8762) centre (0, 0) ccw
  arc A132 (-10.1095, 16.8762) -> (-10.2067, 16.5541) centre (-9.981, 16.6617) ccw
  arc A133 (-10.0811, 16.16) -> (-10.2067, 16.5541) centre (-11.5787, 15.8999) ccw
  arc A134 (-11.3599, 15.2882) -> (-10.0811, 16.16) centre (-10.9186, 16.0146) ccw
  arc A135 (-11.6809, 15.549) -> (-11.3599, 15.2882) centre (-10.5707, 16.5872) ccw
  arc A136 (-11.6809, 15.549) -> (-12.0162, 15.5762) centre (-11.8635, 15.3783) ccw
  arc A137 (-12.0162, 15.5762) -> (-12.5118, 15.181) centre (0, 0) ccw
  arc A138 (-12.5118, 15.181) -> (-12.5599, 14.848) centre (-12.3528, 14.9881) ccw
  arc A139 (-12.377, 14.477) -> (-12.5599, 14.848) centre (-13.8191, 13.9966) ccw
  arc A140 (-13.5116, 13.4243) -> (-12.377, 14.477) centre (-13.1835, 14.2084) ccw
  arc A141 (-13.8679, 13.6344) -> (-13.5116, 13.4243) centre (-12.9248, 14.8264) ccw
  arc A142 (-13.8679, 13.6344) -> (-14.2035, 13.6113) centre (-14.023, 13.4384) ccw
  arc A143 (-14.2035, 13.6113) -> (-14.6347, 13.1466) centre (0, 0) ccw
  arc A144 (-14.6347, 13.1466) -> (-14.6326, 12.8102) centre (-14.4487, 12.9796) ccw
  arc A145 (-14.3965, 12.4706) -> (-14.6326, 12.8102) centre (-15.7509, 11.7807) ccw
  arc A146 (-15.3615, 11.2606) -> (-14.3965, 12.4706) centre (-15.1539, 12.0848) ccw
  arc A147 (-15.7451, 11.4152) -> (-15.3615, 11.2606) centre (-14.9902, 12.7345) ccw
  arc A148 (-15.7451, 11.4152) -> (-16.0735, 11.3424) centre (-15.8693, 11.1982) ccw
  arc A149 (-16.0735, 11.3424) -> (-16.4306, 10.8186) centre (0, 0) ccw
  arc A150 (-16.4306, 10.8186) -> (-16.3785, 10.4863) centre (-16.2218, 10.6811) ccw
  arc A151 (-16.0943, 10.1857) -> (-16.3785, 10.4863) centre (-17.3308, 9.3015) ccw
  arc A152 (-16.8682, 8.8453) -> (-16.0943, 10.1857) centre (-16.7858, 9.6913) ccw
  arc A153 (-17.2706, 8.941) -> (-16.8682, 8.8453) centre (-16.7208, 10.3581) ccw
  arc A154 (-17.2706, 8.941) -> (-17.5845, 8.8201) centre (-17.361, 8.708) ccw
  arc A155 (-17.5845, 8.8201) -> (-17.8596, 8.2489) centre (0, 0) ccw
  arc A156 (-17.8596, 8.2489) -> (-17.7584, 7.9281) centre (-17.6326, 8.1441) ccw
  arc A157 (-17.4327, 7.6732) -> (-17.7584, 7.9281) centre (-18.5235, 6.6146) ccw
  arc A158 (-17.9981, 6.2324) -> (-17.4327, 7.6732) centre (-18.0427, 7.0812) ccw
  arc A159 (-18.4103, 6.2671) -> (-17.9981, 6.2324) centre (-18.0778, 7.7503) ccw
  arc A160 (-18.4103, 6.2671) -> (-18.7027, 6.1007) centre (-18.465, 6.0232) ccw
  arc A161 (-18.7027, 6.1007) -> (-18.8895, 5.4949) centre (0, 0) ccw
  arc A162 (-18.8895, 5.4949) -> (-18.7417, 5.1927) centre (-18.6495, 5.4251) ccw
  arc A163 (-18.3816, 4.9893) -> (-18.7417, 5.1927) centre (-19.3025, 3.78) ccw
  arc A164 (-18.726, 3.4803) -> (-18.3816, 4.9893) centre (-18.8966, 4.313) ccw
  arc A165 (-19.1387, 3.4532) -> (-18.726, 3.4803) centre (-19.031, 4.9694) ccw
  arc A166 (-19.1387, 3.4532) -> (-19.403, 3.2451) centre (-19.1565, 3.2038) ccw
  arc A167 (-19.403, 3.2451) -> (-19.4975, 2.6182) centre (0, 0) ccw
  arc A168 (-19.4975, 2.6182) -> (-19.3063, 2.3414) centre (-19.2497, 2.585) ccw
  arc A169 (-18.9199, 2.1939) -> (-19.3063, 2.3414) centre (-19.6503, 0.8609) ccw
  arc A170 (-19.0356, 0.6505) -> (-18.9199, 2.1939) centre (-19.3283, 1.4485) ccw
  arc A171 (-19.4396, 0.5622) -> (-19.0356, 0.6505) centre (-19.5591, 2.0775) ccw
  arc A172 (-19.4396, 0.5622) -> (-19.67, 0.317) centre (-19.42, 0.3129) ccw
  arc A173 (-19.67, 0.317) -> (-19.67, -0.317) centre (0, 0) ccw
  arc A174 (-19.67, -0.317) -> (-19.4396, -0.5622) centre (-19.42, -0.3129) ccw
  arc A175 (-19.0356, -0.6505) -> (-19.4396, -0.5622) centre (-19.5591, -2.0775) ccw
  arc A176 (-18.9199, -2.1939) -> (-19.0356, -0.6505) centre (-19.3283, -1.4485) ccw
  arc A177 (-19.3063, -2.3414) -> (-18.9199, -2.1939) centre (-19.6503, -0.8609) ccw
  arc A178 (-19.3063, -2.3414) -> (-19.4975, -2.6182) centre (-19.2497, -2.585) ccw
  arc A179 (-19.4975, -2.6182) -> (-19.403, -3.2451) centre (0, 0) ccw
  arc A180 (-19.403, -3.2451) -> (-19.1387, -3.4532) centre (-19.1565, -3.2038) ccw
  arc A181 (-18.726, -3.4803) -> (-19.1387, -3.4532) centre (-19.031, -4.9694) ccw
  arc A182 (-18.3816, -4.9893) -> (-18.726, -3.4803) centre (-18.8966, -4.313) ccw
  arc A183 (-18.7417, -5.1927) -> (-18.3816, -4.9893) centre (-19.3025, -3.78) ccw
  arc A184 (-18.7417, -5.1927) -> (-18.8895, -5.4949) centre (-18.6495, -5.4251) ccw
  arc A185 (-18.8895, -5.4949) -> (-18.7027, -6.1007) centre (0, 0) ccw
  arc A186 (-18.7027, -6.1007) -> (-18.4103, -6.2671) centre (-18.465, -6.0232) ccw
  arc A187 (-17.9981, -6.2324) -> (-18.4103, -6.2671) centre (-18.0778, -7.7503) ccw
  arc A188 (-17.4327, -7.6732) -> (-17.9981, -6.2324) centre (-18.0427, -7.0812) ccw
  arc A189 (-17.7584, -7.9281) -> (-17.4327, -7.6732) centre (-18.5235, -6.6146) ccw
  arc A190 (-17.7584, -7.9281) -> (-17.8596, -8.2489) centre (-17.6326, -8.1441) ccw
  arc A191 (-17.8596, -8.2489) -> (-17.5845, -8.8201) centre (0, 0) ccw
  arc A192 (-17.5845, -8.8201) -> (-17.2706, -8.941) centre (-17.361, -8.708) ccw
  arc A193 (-16.8682, -8.8453) -> (-17.2706, -8.941) centre (-16.7208, -10.3581) ccw
  arc A194 (-16.0943, -10.1857) -> (-16.8682, -8.8453) centre (-16.7858, -9.6913) ccw
  arc A195 (-16.3785, -10.4863) -> (-16.0943, -10.1857) centre (-17.3308, -9.3015) ccw
  arc A196 (-16.3785, -10.4863) -> (-16.4306, -10.8186) centre (-16.2218, -10.6811) ccw
  arc A197 (-16.4306, -10.8186) -> (-16.0735, -11.3424) centre (0, 0) ccw
  arc A198 (-16.0735, -11.3424) -> (-15.7451, -11.4152) centre (-15.8693, -11.1982) ccw
  arc A199 (-15.3615, -11.2606) -> (-15.7451, -11.4152) centre (-14.9902, -12.7345) ccw
  arc A200 (-14.3965, -12.4706) -> (-15.3615, -11.2606) centre (-15.1539, -12.0848) ccw
  arc A201 (-14.6326, -12.8102) -> (-14.3965, -12.4706) centre (-15.7509, -11.7807) ccw
  arc A202 (-14.6326, -12.8102) -> (-14.6347, -13.1466) centre (-14.4487, -12.9796) ccw
  arc A203 (-14.6347, -13.1466) -> (-14.2035, -13.6113) centre (0, 0) ccw
  arc A204 (-14.2035, -13.6113) -> (-13.8679, -13.6344) centre (-14.023, -13.4384) ccw
  arc A205 (-13.5116, -13.4243) -> (-13.8679, -13.6344) centre (-12.9248, -14.8264) ccw
  arc A206 (-12.377, -14.477) -> (-13.5116, -13.4243) centre (-13.1835, -14.2084) ccw
  arc A207 (-12.5599, -14.848) -> (-12.377, -14.477) centre (-13.8191, -13.9966) ccw
  arc A208 (-12.5599, -14.848) -> (-12.5118, -15.181) centre (-12.3528, -14.9881) ccw
  arc A209 (-12.5118, -15.181) -> (-12.0162, -15.5762) centre (0, 0) ccw
  arc A210 (-12.0162, -15.5762) -> (-11.6809, -15.549) centre (-11.8635, -15.3783) ccw
  arc A211 (-11.3599, -15.2882) -> (-11.6809, -15.549) centre (-10.5707, -16.5872) ccw
  arc A212 (-10.0811, -16.16) -> (-11.3599, -15.2882) centre (-10.9186, -16.0146) ccw
  arc A213 (-10.2067, -16.5541) -> (-10.0811, -16.16) centre (-11.5787, -15.8999) ccw
  arc A214 (-10.2067, -16.5541) -> (-10.1095, -16.8762) centre (-9.981, -16.6617) ccw
  arc A215 (-10.1095, -16.8762) -> (-9.5605, -17.1932) centre (0, 0) ccw
  arc A216 (-9.5605, -17.1932) -> (-9.233, -17.1163) centre (-9.439, -16.9747) ccw
  arc A217 (-8.9545, -16.8105) -> (-9.233, -17.1163) centre (-7.9804, -17.9774) ccw
  arc A218 (-7.56, -17.4821) -> (-8.9545, -16.8105) centre (-8.4098, -17.463) ccw
  arc A219 (-7.6254, -17.8905) -> (-7.56, -17.4821) centre (-9.0796, -17.4481) ccw
  arc A220 (-7.6254, -17.8905) -> (-7.4813, -18.1945) centre (-7.3862, -17.9632) ccw
  arc A221 (-7.4813, -18.1945) -> (-6.8912, -18.4261) centre (0, 0) ccw
  arc A222 (-6.8912, -18.4261) -> (-6.5788, -18.3012) centre (-6.8036, -18.1919) ccw
  arc A223 (-6.349, -17.9573) -> (-6.5788, -18.3012) centre (-5.2119, -18.966) ccw
  arc A224 (-4.87, -18.4136) -> (-6.349, -17.9573) centre (-5.7131, -18.5214) ccw
  arc A225 (-4.8738, -18.8272) -> (-4.87, -18.4136) centre (-6.3777, -18.6064) ccw
  arc A226 (-4.8738, -18.8272) -> (-4.686, -19.1063) centre (-4.6264, -18.8635) ccw
  arc A227 (-4.686, -19.1063) -> (-4.068, -19.2473) centre (0, 0) ccw
  arc A228 (-4.068, -19.2473) -> (-3.7777, -19.0773) centre (-4.0163, -19.0027) ccw
  arc A229 (-3.6017, -18.703) -> (-3.7777, -19.0773) centre (-2.3269, -19.531) ccw
  arc A230 (-2.0712, -18.9337) -> (-3.6017, -18.703) centre (-2.8888, -19.166) ccw
  arc A231 (-2.0133, -19.3433) -> (-2.0712, -18.9337) centre (-3.5333, -19.3492) ccw
  arc A232 (-2.0133, -19.3433) -> (-1.786, -19.5913) centre (-1.7633, -19.3423) ccw
  arc A233 (-1.786, -19.5913) -> (-1.1539, -19.6387) centre (0, 0) ccw
  arc A234 (-1.1539, -19.6387) -> (-0.8921, -19.4273) centre (-1.1392, -19.3891) ccw
  arc A235 (-0.7739, -19.0309) -> (-0.8921, -19.4273) centre (0.61, -19.6597) ccw
  arc A236 (0.7739, -19.0309) -> (-0.7739, -19.0309) centre (0, -19.3825) ccw
  arc A237 (0.8921, -19.4273) -> (0.7739, -19.0309) centre (-0.61, -19.6597) ccw
  arc A238 (0.8921, -19.4273) -> (1.1539, -19.6387) centre (1.1392, -19.3891) ccw
  arc A239 (1.1539, -19.6387) -> (1.786, -19.5913) centre (0, 0) ccw
  circle A240 centre (0, 0) radius 20.6725
  arc A241 (1.786, -19.5913) -> (2.0133, -19.3433) centre (1.7633, -19.3423) ccw
  arc A242 (2.0712, -18.9337) -> (2.0133, -19.3433) centre (3.5333, -19.3492) ccw
  arc A243 (3.6017, -18.703) -> (2.0712, -18.9337) centre (2.8888, -19.166) ccw
  arc A244 (3.7777, -19.0773) -> (3.6017, -18.703) centre (2.3269, -19.531) ccw
  arc A245 (3.7777, -19.0773) -> (4.068, -19.2473) centre (4.0163, -19.0027) ccw
  arc A246 (4.068, -19.2473) -> (4.686, -19.1063) centre (0, 0) ccw
  arc A247 (4.686, -19.1063) -> (4.8738, -18.8272) centre (4.6264, -18.8635) ccw
  arc A248 (4.87, -18.4136) -> (4.8738, -18.8272) centre (6.3777, -18.6064) ccw
  arc A249 (6.349, -17.9573) -> (4.87, -18.4136) centre (5.7131, -18.5214) ccw
  arc A250 (6.5788, -18.3012) -> (6.349, -17.9573) centre (5.2119, -18.966) ccw
  arc A251 (6.5788, -18.3012) -> (6.8912, -18.4261) centre (6.8036, -18.1919) ccw
  arc A252 (6.8912, -18.4261) -> (7.4813, -18.1945) centre (0, 0) ccw
  dimension "d33" = 41.345
  measures "d33" diameter of A240
extrude "Extrusion3" add sketch "Skizze3" along normal blind 1 contours A0 A1 A2 A3 A4 A5 A6 A7 A8 A9 A10 A11 A12 A13 A14 A15 A16 A17 A18 A19 A20 A21 A22 A23 A24 A25 A26 A27 A28 A29 A30 A31 A32 A33 A34 A35 A36 A37 A38 A39 A40 A41 A42 A43 A44 A45 A46 A47 A48 A49 A50 A51 A52 A53 A54 A55 A56 A57 A58 A59 A60 A61 A62 A63 A64 A65 A66 A67 A68 A69 A70 A71 A72 A73 A74 A75 A76 A77 A78 A79 A80 A81 A82 A83 A84 A85 A86 A87 A88 A89 A90 A91 A92 A93 A94 A95 A96 A97 A98 A99 A100 A101 A102 A103 A104 A105 A106 A107 A108 A109 A110 A111 A112 A113 A114 A115 A116 A117 A118 A119 A120 A121 A122 A123 A124 A125 A126 A127 A128 A129 A130 A131 A132 A133 A134 A135 A136 A137 A138 A139 A140 A141 A142 A143 A144 A145 A146 A147 A148 A149 A150 A151 A152 A153 A154 A155 A156 A157 A158 A159 A160 A161 A162 A163 A164 A165 A166 A167 A168 A169 A170 A171 A172 A173 A174 A175 A176 A177 A178 A179 A180 A181 A182 A183 A184 A185 A186 A187 A188 A189 A190 A191 A192 A193 A194 A195 A196 A197 A198 A199 A200 A201 A202 A203 A204 A205 A206 A207 A208 A209 A210 A211 A212 A213 A214 A215 A216 A217 A218 A219 A220 A221 A222 A223 A224 A225 A226 A227 A228 A229 A230 A231 A232 A233 A234 A235 A236 A237 A238 A239 A241 A242 A243 A244 A245 A246 A247 A248 A249 A250 A251 A252 | A240 bodies 1
sketch "Skizze16" plane through (0, 8, 0) normal (0, 1, 0) x (-1, 0, 0)
  circle A0 centre (0, 0) radius 19.7176
  line L0 (3.7528, -6.5) -> (7.5056, 0)
  line L1 (7.5056, 0) -> (3.7528, 6.5)
  line L2 (3.7528, 6.5) -> (-3.7528, 6.5)
  line L3 (-3.7528, 6.5) -> (-7.5056, 0)
  line L4 (-7.5056, 0) -> (-3.7528, -6.5)
  line L5 (-3.7528, -6.5) -> (3.7528, -6.5)
  circle A1 centre (0, 0) radius 3.5
  circle A2 centre (0, 0) radius 16.0986
  circle A3 centre (0, 0) radius 20.6725
  dimension "d110" = 13
  dimension "d111" = 7
  measures "d110" distance of L1 L4
  measures "d111" diameter of A1